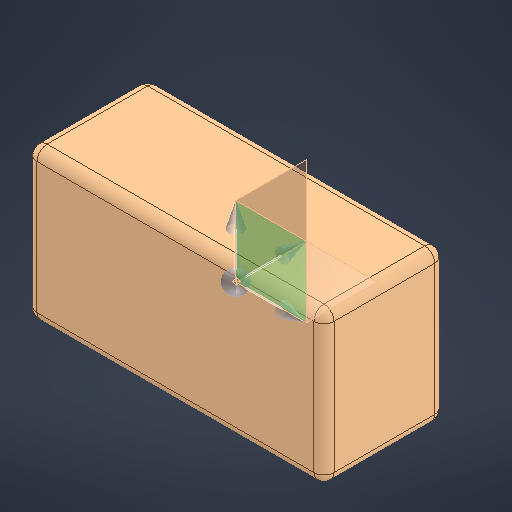
# Autodesk Inventor part: P_Akku_Dummy
Saved by Autodesk Inventor 2026 (Build 300175000, 175)
## iProperties
Created: 2025-08-24
Part Number: P_Akku_Dummy
Material: Generisch
Document SubType Name: Modeling
Designer: FAL
Density: 3.18269 g/cm^3
Appearance: Vorgabe
Mass: 134 g
Surface Area: 74.1947 cm^2
Volume: 42.1027 cm^3
Author: FAL
Autodesk Inventor part; units mm, degrees
ref_plane "YZ Plane" through (0, 0, 0) normal (1, 0, 0) x (0, 1, 0)
ref_plane "XZ Plane" through (0, 0, 0) normal (0, 1, 0) x (-1, 0, 0)
ref_plane "XY Plane" through (0, 0, 0) normal (0, 0, 1) x (1, 0, 0)
sketch "Skizze1" plane through (0, 0, 0) normal (0, 0, 1) x (1, 0, 0)
  line L0 (29.5, -12) -> (-29.5, -12)
  line L1 (-29.5, -12) -> (-29.5, 12)
  line L2 (-29.5, 12) -> (29.5, 12)
  line L3 (29.5, 12) -> (29.5, -12)
  line L4 (29.5, -12) -> (-29.5, 12) construction
  line L5 (-29.5, -12) -> (29.5, 12) construction
  point P0 (0, 0)
  dimension "d0" = 59
  dimension "d1" = 24
  constraints: 12 end point, 2 midpoint, 2 parallel, 1 horizontal, 1 perpendicular
  measures "d0" distance of L1.end L2.end
  measures "d1" distance of L2.end L0.start
extrude "Extrusion1" add sketch "Skizze1" along normal mid plane 30
fillet "Rundung1" radius 2 4 edges at (-29.5, -12, 0) (29.5, -12, 0) (-29.5, 12, 0) (29.5, 12, 0)
fillet "Rundung2" radius 2 16 edges at (28.9142, -11.4142, 15) (29.5, 0, 15) (28.9142, 11.4142, 15) (0, 12, 15) (-28.9142, 11.4142, 15) (-29.5, 0, 15) (-28.9142, -11.4142, 15) (0, -12, 15) (-28.9142, -11.4142, -15) (-29.5, 0, -15) (-28.9142, 11.4142, -15) (0, 12, -15) (28.9142, 11.4142, -15) (29.5, 0, -15) (28.9142, -11.4142, -15) (0, -12, -15)
